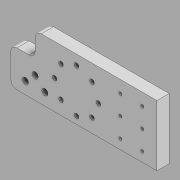
# Autodesk Inventor part: A01209499_13PT
Saved by Autodesk Inventor 2020 (Build 240168000, 168)
## iProperties
Created: 2019-11-28
Part Number: A01209499_13PT
Material: Generic
Document SubType Name: Modeling
Designer: Jorge
Density: 1 g/cm^3
Appearance: Default
Author: Jorge
Autodesk Inventor part; units mm, degrees
ref_plane "YZ Plane" through (0, 0, 0) normal (1, 0, 0) x (0, 1, 0)
ref_plane "XZ Plane" through (0, 0, 0) normal (0, 1, 0) x (-1, 0, 0)
ref_plane "XY Plane" through (0, 0, 0) normal (0, 0, 1) x (1, 0, 0)
sketch "Sketch1" plane through (0, 0, 0) normal (0, 0, 1) x (1, 0, 0)
  line L0 (0, 0) -> (0, 38.1)
  line L1 (0, 38.1) -> (25.4, 38.1)
  line L2 (25.4, 38.1) -> (25.4, 63.5)
  line L3 (25.4, 63.5) -> (152.4, 63.5)
  line L4 (152.4, 63.5) -> (152.4, 0)
  line L5 (152.4, 0) -> (0, 0)
  dimension "d0" = 152.4
  dimension "d1" = 63.5
  dimension "d2" = 127
  dimension "d3" = 38.1
  constraints: 12 end point, 5 perpendicular, 1 vertical
  measures "d0" distance of L4.end L0.start
  measures "d1" distance between parallel lines of L5 L3
  measures "d2" distance of L2.end L3.end
  measures "d3" distance between parallel lines of L5 L1
extrude "Extrusion1" add sketch "Sketch1" along normal blind 12.7
sketch "Sketch2" plane through (0, 0, 12.7) normal (0, 0, 1) x (1, 0, 0)
  line L0 (152.4, 0) -> (152.4, 63.5) projected
  line L1 (15.24, 12.7) -> (35.56, 12.7) construction
  line L2 (0, 0) -> (152.4, 0) construction
  point P0 (25.4, 22.86)
  dimension "d6" = 127
  dimension "d7" = 10.16
  dimension "d8" = 12.7
  dimension "d9" = 10.16
  dimension "d10" = 10.16
  constraints: 2 end point, 1 horizontal
  measures "d6" distance from line of L0 point (25.4, 22.86)
  measures "d7" horizontal distance of L1.start point (25.4, 22.86)
  measures "d8" distance between parallel lines of L2 L1
  measures "d9" horizontal distance of point (25.4, 22.86) L1.start
  measures "d10" horizontal distance of L1.end point (25.4, 22.86)
hole "Hole1" at (25.4, 22.86, 12.7) at (15.24, 12.7, 12.7) at (35.56, 12.7, 12.7) direction (0, 0, -1) diameter 6.35 end through all
sketch "Sketch3" plane through (0, 0, 12.7) normal (0, 0, 1) x (1, 0, 0)
  circle A0 centre (68.58, 30.48) radius 22.86 construction
  line L0 (152.4, 0) -> (152.4, 63.5) construction
  line L1 (0, 0) -> (152.4, 0) construction
  line L2 (68.58, 30.48) -> (68.58, 55.3501) construction
  point P0 (68.58, 53.34)
  dimension "d18" = 45.72
  dimension "d19" = 83.82
  dimension "d20" = 30.48
  constraints: 2 end point, 1 coincident, 1 point on line, 1 vertical, 1 vertical alignment, 2 other
  measures "d19" distance from line of L0 point (68.58, 30.48)
  measures "d20" distance from line of L1 point (68.58, 30.48)
hole "Hole2" at (68.58, 53.34, 12.7) direction (0, 0, -1) diameter 4.7752 end through all
pattern_circular "Circular Pattern1" count 8 over 360 about axis through (68.58, 30.48, 12.7) along (0, 0, 1) of "Hole2"
sketch "Sketch4" plane through (0, 0, 12.7) normal (0, 0, 1) x (1, 0, 0)
  line L0 (152.4, 0) -> (152.4, 63.5) construction
  line L1 (0, 0) -> (152.4, 0) projected
  point P0 (114.3, 50.8)
  dimension "d32" = 38.1
  dimension "d37" = 50.8
  measures "d32" distance from line of L0 point (114.3, 50.8)
  measures "d37" distance from line of L1 point (114.3, 50.8)
hole "Hole3" at (114.3, 50.8, 12.7) direction (0, 0, -1) diameter 3.175 end through all
pattern_linear "Rectangular Pattern1" count 2 spacing 22.86 along (1, 0, 0) count 3 spacing 20.32 along (0, -1, 0) of "Hole3"
fillet "Fillet1" radius 6.35 4 edges at (25.4, 38.1, 6.35) (0, 38.1, 6.35) (25.4, 63.5, 6.35) (0, 0, 6.35)
body "Solid1"
